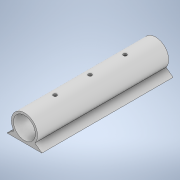
# Autodesk Inventor part: Pin Cylinder
Saved by Autodesk Inventor 2022 (Build 260153000, 153)
## iProperties
Created: 2022-03-17
Part Number: Pin Cylinder
Material: Generic
Document SubType Name: Modeling
Designer: Alexa
Density: 1 g/cm^3
Appearance: Default
Author: Alexa
Autodesk Inventor part; units mm, degrees
ref_plane "YZ Plane" through (0, 0, 0) normal (1, 0, 0) x (0, 1, 0)
ref_plane "XZ Plane" through (0, 0, 0) normal (0, 1, 0) x (-1, 0, 0)
ref_plane "XY Plane" through (0, 0, 0) normal (0, 0, 1) x (1, 0, 0)
sketch "Sketch1" plane through (0, 0, 0) normal (0, 1, 0) x (-1, 0, 0)
  line L0 (0, 0) -> (60, 0)
  line L1 (60, 0) -> (60, -150)
  line L2 (60, -150) -> (0, -150)
  line L3 (0, -150) -> (0, 0)
  line L4 (0, 0) -> (40, 0)
  line L5 (40, 0) -> (40, -150)
  line L6 (40, -150) -> (0, -150)
  line L7 (0, -150) -> (0, 0)
  dimension "d0" = 60
  dimension "d1" = 150
  dimension "d2" = 40
  constraints: 16 end point, 4 parallel, 2 horizontal, 2 perpendicular, 1 point on line
  measures "d0" distance of L1.end L2.end
  measures "d1" distance of L0.end L1.end
  measures "d2" distance of L5.end L6.end
extrude "Extrusion1" add sketch "Sketch1" along normal blind 30 contours L0 L5 L2 L3
sketch "Sketch2" plane through (0, 30, 0) normal (0, 1, 0) x (1, 0, 0)
  line L0 (0, 150) -> (-40, 150) projected
  line L1 (-20, 150) -> (-20, 0)
  line L2 (-20, 0) -> (-20, 75)
  line L3 (-20, 75) -> (-20, 150)
  line L4 (-20, 75) -> (-20, 115)
  line L5 (-20, 75) -> (-20, 35)
  line L6 (-20, 35) -> (-20, 115)
  circle A0 centre (-20, 35) radius 1.65
  circle A1 centre (-20, 75) radius 1.75
  circle A2 centre (-20, 35) radius 1.75
  circle A3 centre (-20, 115) radius 1.75
  circle A4 centre (-20, 35) radius 2
  circle A5 centre (-20, 75) radius 2
  circle A6 centre (-20, 115) radius 2
  point P0 (0, 0)
  dimension "d5" = 40
  dimension "d6" = 40
  dimension "d7" = 3.3
  dimension "d8" = 3.5
  dimension "d9" = 3.5
  dimension "d10" = 3.5
  dimension "d11" = 4
  dimension "d12" = 4
  dimension "d13" = 4
  constraints: 12 end point, 7 centre point, 7 coincident, 2 collinear, 2 midpoint, 2 point on line, 1 vertical
  measures "d5" distance of L2.end L4.end
  measures "d6" distance of L2.end L5.end
  measures "d7" diameter of A0
  measures "d8" diameter of A1
  measures "d9" diameter of A2
  measures "d10" diameter of A3
  measures "d11" diameter of A4
  measures "d12" diameter of A5
  measures "d13" diameter of A6
extrude "Extrusion2" cut sketch "Sketch2" against normal blind 4
sketch "Sketch3" plane through (-40, 0, 0) normal (0, 0, 1) x (1, 0, 0)
  line L0 (0, 0) -> (0, 30) projected
  line L1 (40, 0) -> (40, 30) projected
  line L2 (0, 30) -> (40, 30)
  line L3 (40, 30) -> (40, 15)
  line L4 (40, 15) -> (0, 15)
  line L5 (0, 15) -> (0, 30)
  line L6 (0, 0) -> (40, 0) projected
  line L7 (40, 15) -> (20, 15)
  line L8 (20, 15) -> (20, 0)
  line L9 (20, 0) -> (40, 0)
  line L10 (40, 0) -> (40, 15)
  circle A0 centre (20, 15) radius 15
  line L11 (0, 0) -> (40, 0)
  line L12 (40, 0) -> (40, -5)
  line L13 (40, -5) -> (0, -5)
  line L14 (0, -5) -> (0, 0)
  circle A1 centre (20, 15) radius 12.5
  line L15 (20, 15) -> (0, 0)
  line L16 (20, 15) -> (40, 0)
  point P0 (20, 30)
  point P1 (32, 6)
  point P2 (8, 6)
  dimension "d16" = 30
  dimension "d17" = 5
  dimension "d18" = 25
  constraints: 28 end point, 6 parallel, 3 horizontal, 3 perpendicular, 2 centre point, 2 coincident, 2 midpoint
  measures "d16" diameter of A0
  measures "d17" distance of L11.end L12.end
  measures "d18" diameter of A1
extrude "Extrusion3" cut sketch "Sketch3" against normal blind 150 contours L0 L4 A0 L15 | L0 L2 A0 L4 | L16 A0 L4 L1 | A1 L15 L8 | L8 L16 A1 | A1 L4 L15 | L2 L1 L4 A0 | A1 L4 | L4 A1 L16
body "Solid1"
